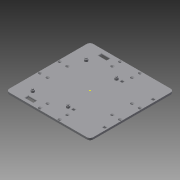
# Autodesk Inventor part: toppart
Saved by Autodesk Inventor 2015 (Build 190159000, 159)
## iProperties
Created: 2015-11-30
Part Number: toppart
Material: Generic
Document SubType Name: Modeling
Designer: Ross
Density: 1 g/cm^3
Appearance: Default
Author: Ross
Autodesk Inventor part; units mm, degrees
sketch "Sketch1" plane through (0, 0, 0) normal (0, 1, 0) x (-1, 0, 0)
  line L0 (0, 65) -> (65, 65)
  line L1 (65, 65) -> (65, -65)
  line L2 (65, -65) -> (0, -65)
  line L3 (0, -65) -> (-65, -65)
  line L4 (-65, -65) -> (-65, 65)
  line L5 (-65, 65) -> (0, 65)
  point P0 (0, 0)
  dimension "d0" = 65
  dimension "d1" = 65
  dimension "d2" = 130
  dimension "d3" = 65
  constraints: 12 end point, 4 perpendicular, 2 point on line
  measures "d0" distance of point (0, 0) L0.start
  measures "d1" distance of L0.start L0.end
  measures "d2" distance of L0.end L1.end
  measures "d3" distance of L2.end L3.end
extrude "Extrusion1" add sketch "Sketch1" along normal blind 3
fillet "Fillet1" radius 5 4 edges at (-65, 1.5, 65) (65, 1.5, 65) (-65, 1.5, -65) (65, 1.5, -65)
sketch "Sketch6" plane through (0, 3, 0) normal (0, 1, 0) x (1, 0, 0)
  line L0 (60, 65) -> (-60, 65) projected
  line L1 (0, 65) -> (-18.3, 65)
  line L2 (-18.3, 65) -> (-18.3, 47)
  line L3 (0, 65) -> (18.3, 65)
  line L4 (18.3, 65) -> (18.3, 47)
  line L5 (18.3, 47) -> (-18.3, 47)
  line L6 (-18.3, 47) -> (-15.3, 47)
  line L7 (-15.3, 47) -> (-15.3, 50)
  line L8 (-15.3, 65) -> (-15.3, 62)
  line L9 (0, 65) -> (0, 47)
  circle A0 centre (-15.3, 62) radius 2.4
  circle A1 centre (-15.3, 50) radius 2.4
  circle A2 centre (15.3, 62) radius 2.4
  circle A3 centre (15.3, 50) radius 2.4
  point P0 (0, 0)
  dimension "d20" = 18.3
  dimension "d21" = 18
  dimension "d22" = 18.3
  dimension "d23" = 3
  dimension "d24" = 3
  dimension "d25" = 3
  dimension "d40" = 4.8
  dimension "d41" = 4.8
  constraints: 18 end point, 4 centre point, 4 point on line, 2 coincident, 2 midpoint, 2 perpendicular, 2 symmetric about line, 1 vertical, 2 other
  measures "d20" distance of L1.start L1.end
  measures "d21" distance of L1.end L2.end
  measures "d22" distance of L1.start L3.end
  measures "d23" distance of L2.end L6.end
  measures "d24" distance of L6.end L7.end
  measures "d25" distance of L8.start L8.end
  measures "d40" diameter of A0
  measures "d41" diameter of A1
extrude "Extrusion6" cut sketch "Sketch6" against normal blind 1.5 contours A0
sketch "Sketch9" plane through (-15.3, 1.5, -62) normal (0, 1, 0) x (1, 0, 0)
  circle A0 centre (0, 0) radius 1.25
  point P0 (15.3, -62)
  dimension "d44" = 2.5
  constraints: 1 centre point
  measures "d44" diameter of A0
extrude "Extrusion7" cut sketch "Sketch9" against normal blind 1.5
ref_plane "Work Plane1" through (-15.25, 0, 0) normal (1, 0, 0) x (0, 1, 0)
sketch "Sketch11" plane through (-15.25, 0, 0) normal (1, 0, 0) x (0, 1, 0)
  line L0 (3, -59.6) -> (3, -64.4) projected
  line L1 (3, -59.6) -> (1.5, -59.6)
  line L2 (1.5, -59.6) -> (1.5, -64.4) projected
  line L3 (3, -59.6) -> (1.5, -59.6) projected
  line L4 (1.5, -59.6) -> (1.5, -60.7474)
  line L5 (1.5, -60.75) -> (1.5, -63.25) projected
  line L6 (1.5, -60.75) -> (3, -59.6)
  point P0 (0, 0)
  constraints: 8 end point, 1 collinear, 1 point on line
sketch3d "3D Sketch1"
  arc A0 (-12.9, 3, -62) -> (-15.3, 3, -59.6) centre (-15.3, 3, -62) ccw
  arc A1 (-15.3, 3, -59.6) -> (-17.7, 3, -62) centre (-15.3, 3, -62) ccw
  arc A2 (-17.7, 3, -62) -> (-15.3, 3, -64.4) centre (-15.3, 3, -62) ccw
  arc A3 (-15.3, 3, -64.4) -> (-12.9, 3, -62) centre (-15.3, 3, -62) ccw
sweep "Sweep1" add profiles "Sketch11" path "3D Sketch1"
ref_plane "Work Plane2" through (60, 0, -56) normal (0, 0, -1) x (-1, 0, 0)
ref_plane "Work Plane3" through (0, 0, -60) normal (-1, 0, 0) x (0, 0, 1)
mirror "Mirror5" about plane through (0, 0, -60) normal (-1, 0, 0) of "Extrusion7", "Sweep1"
mirror "Mirror6" about plane through (0, 0, -60) normal (-1, 0, 0) of "Extrusion6", "Extrusion7", "Sweep1"
mirror "Mirror7" about plane through (60, 0, -56) normal (0, 0, -1) of "Extrusion6", "Extrusion7", "Sweep1", "Mirror6"
pattern_circular "Circular Pattern3" count 4 over 360 about axis through (0, -10, 0) along (0, 1, 0) of "Extrusion6", "Extrusion7", "Sweep1", "Mirror6", "Mirror7"
sketch "Sketch14" plane through (0, 3, 0) normal (0, 1, 0) x (1, 0, 0)
  line L0 (65, -60) -> (10, -60)
  line L1 (10, -60) -> (10, 65)
  line L2 (-60, 65) -> (60, 65) projected
  line L3 (10, -60) -> (-44, -60)
  line L4 (-44, -60) -> (-44, 65)
  line L5 (37.5, -60) -> (37.5, 65)
  line L6 (37.5, -60) -> (14.5, -60)
  line L7 (14.5, -60) -> (14.5, 65)
  line L8 (60.5, -60) -> (60.5, 65)
  line L9 (65, -60) -> (65, 60) projected
  line L10 (59, -39.0209) -> (62, -39.0209)
  line L11 (62, -39.0209) -> (59, -39.0209)
  line L12 (59, -39.0209) -> (59, -36.0209)
  line L13 (59, -36.0209) -> (62, -36.0209)
  line L14 (62, -36.0209) -> (62, -39.0209)
  point P0 (0, 0)
  dimension "d56" = 55
  dimension "d57" = 54
  dimension "d58" = 23
  dimension "d63" = 3
  dimension "d64" = 3
  constraints: 26 end point, 5 point on line, 4 perpendicular, 3 horizontal, 2 parallel, 2 symmetric about line, 1 midpoint, 1 vertical
  measures "d56" distance of L0.start L0.end
  measures "d57" distance of L0.end L3.end
  measures "d58" distance of L5.start L6.end
  measures "d63" distance of L12.end L13.end
  measures "d64" distance of L11.end L12.end
extrude "Extrusion8" cut sketch "Sketch14" against normal blind 3 contours L10 L12 L13 L8 | L8 L13 L14 L10
fillet "Fillet2" radius 1 4 edges at (62, 3, 37.5209) (60.5, 3, 39.0209) (59, 3, 37.5209) (60.5, 3, 36.0209)
fillet "Fillet3" radius 2 1 edges at (59, 0, 37.5209)
ref_plane "Work Plane4" through (36.5, 0, -60) normal (-1, 0, 0) x (0, 0, 1)
mirror "Mirror8" about plane through (36.5, 0, -60) normal (-1, 0, 0) of "Extrusion8", "Fillet2", "Fillet3"
sketch "Sketch15" plane through (0, 3, 0) normal (0, 1, 0) x (1, 0, 0)
  point P0 (0, 0)
mirror "Mirror9" about plane through (0, 0, 0) normal (0, 0, 1) of "Fillet2", "Extrusion8", "Fillet3", "Mirror8"
sketch "Sketch16" plane through (0, 3, 0) normal (0, 1, 0) x (1, 0, 0)
  line L0 (63, -60) -> (11, -60)
  line L1 (11, -60) -> (11, 53.4976)
  line L2 (11, 53.4976) -> (63, 53.4976)
  line L3 (63, 53.4976) -> (63, -60)
  line L4 (9.645, 0) -> (9.645, -52)
  line L5 (9.645, -52) -> (-44.355, -52)
  line L6 (-44.355, -52) -> (-44.355, 50)
  line L7 (-44.355, 50) -> (9.645, 50)
  line L8 (9.645, 50) -> (9.645, -52)
  line L9 (-40.3154, -54.1219) -> (-28.3154, -54.1219)
  line L10 (-28.3154, -54.1219) -> (-28.3154, -59.1219)
  line L11 (-28.3154, -59.1219) -> (-40.3154, -59.1219)
  line L12 (-40.3154, -59.1219) -> (-40.3154, -54.1219)
  point P0 (0, 0)
  dimension "d70" = 52
  dimension "d71" = 52
  dimension "d72" = 54
  dimension "d73" = 102
  dimension "d74" = 12
  dimension "d75" = 5
  constraints: 26 end point, 6 parallel, 3 horizontal, 3 perpendicular, 1 vertical
  measures "d70" distance of L1.end L2.end
  measures "d71" distance of L4.start L4.end
  measures "d72" distance of L6.end L7.end
  measures "d73" distance of L5.end L6.end
  measures "d74" distance of L10.end L11.end
  measures "d75" distance of L9.end L10.end
extrude "Extrusion9" cut sketch "Sketch16" against normal blind 3 contours L9 L10 L11 L12
fillet "Fillet4" radius 1.5 4 edges at (-34.3154, 3, 59.1219) (-34.3154, 3, 54.1219) (-40.3154, 3, 56.6219) (-28.3154, 3, 56.6219)
fillet "Fillet5" radius 1.5 4 edges at (-34.3154, 0, 54.1219) (-28.3154, 0, 56.6219) (-34.3154, 0, 59.1219) (-40.3154, 0, 56.6219)
mirror "Mirror10" about plane through (0, 0, 0) normal (0, 0, 1) of "Extrusion9", "Fillet4", "Fillet5"
sketch "Sketch17" plane through (0, 3, 0) normal (0, 1, 0) x (1, 0, 0)
  line L0 (0, 0) -> (8, 0)
  line L1 (8, 0) -> (8, -50.76)
  line L2 (8, 0) -> (8, 50.76)
  line L3 (8, 50.76) -> (-45.3, 50.76)
  line L4 (-45.3, 50.76) -> (-45.3, -50.76)
  line L5 (-45.3, -50.76) -> (8, -50.76)
  line L6 (8, 50.76) -> (8, 35.52)
  line L7 (8, 35.52) -> (5.46, 35.52)
  circle A0 centre (5.46, 35.52) radius 2.5
  line L8 (-45.3, 50.76) -> (-45.3, 36.79)
  line L9 (-45.3, 36.79) -> (-42.76, 36.79)
  circle A1 centre (-42.76, 36.79) radius 2.5
  line L10 (8, 50.76) -> (8, -39.41)
  line L11 (8, -39.41) -> (5.46, -39.41)
  circle A2 centre (5.46, -39.41) radius 2.5
  line L12 (-45.3, 50.76) -> (-45.3, -45.76)
  line L13 (-45.3, -45.76) -> (-42.76, -45.76)
  circle A3 centre (-42.76, -45.76) radius 2.5
  dimension "d80" = 8
  dimension "d81" = 50.76
  dimension "d82" = 50.76
  dimension "d83" = 53.3
  dimension "d84" = 15.24
  dimension "d85" = 2.54
  dimension "d86" = 5
  dimension "d87" = 13.97
  dimension "d88" = 2.54
  dimension "d89" = 5
  dimension "d90" = 90.17
  dimension "d91" = 2.54
  dimension "d92" = 5
  dimension "d93" = 96.52
  dimension "d94" = 2.54
  dimension "d95" = 5
  constraints: 28 end point, 6 perpendicular, 4 centre point, 4 coincident, 4 point on line, 2 vertical, 1 horizontal, 1 parallel
  measures "d80" distance of L0.start L0.end
  measures "d81" distance of L0.end L1.end
  measures "d82" distance of L0.end L2.end
  measures "d83" distance of L2.end L3.end
  measures "d84" distance of L2.end L6.end
  measures "d85" distance of L6.end L7.end
  measures "d86" diameter of A0
  measures "d87" distance of L3.end L8.end
  measures "d88" distance of L8.end L9.end
  measures "d89" diameter of A1
  measures "d90" distance of L2.end L10.end
  measures "d91" distance of L10.end L11.end
  measures "d92" diameter of A2
  measures "d93" distance of L3.end L12.end
  measures "d94" distance of L12.end L13.end
  measures "d95" diameter of A3
extrude "Extrusion10" add sketch "Sketch17" along normal blind 3 contours A0 | A1 | A2 | A3
sketch "Sketch18" plane through (-42.76, 6, -36.79) normal (0, 1, 0) x (1, 0, 0)
  circle A0 centre (0, 0) radius 2.5 projected
  circle A1 centre (0, 0) radius 1.5
  point P0 (42.76, -36.79)
  dimension "d98" = 3
  constraints: 1 centre point, 1 coincident
  measures "d98" diameter of A1
extrude "Extrusion11" add sketch "Sketch18" along normal blind 1.5 contours A1
sketch "Sketch19" plane through (5.46, 6, -35.52) normal (0, 1, 0) x (1, 0, 0)
  circle A0 centre (0, 0) radius 2.5 projected
  circle A1 centre (0, 0) radius 1.5
  point P0 (-5.46, -35.52)
  dimension "d101" = 3
  constraints: 1 centre point, 1 coincident
  measures "d101" diameter of A1
extrude "Extrusion12" add sketch "Sketch19" along normal blind 1.5 contours A1
sketch "Sketch20" plane through (5.46, 6, 39.41) normal (0, 1, 0) x (1, 0, 0)
  circle A0 centre (0, 0) radius 1.5
  point P0 (-5.46, 39.41)
  dimension "d104" = 3
  constraints: 1 centre point
  measures "d104" diameter of A0
extrude "Extrusion13" add sketch "Sketch20" along normal blind 1.5
sketch "Sketch21" plane through (-42.76, 6, 45.76) normal (0, 1, 0) x (1, 0, 0)
  circle A0 centre (0, 0) radius 1.5
  point P0 (42.76, 45.76)
  dimension "d107" = 3
  constraints: 1 centre point
  measures "d107" diameter of A0
extrude "Extrusion14" add sketch "Sketch21" along normal blind 1.5
fillet "Fillet6" radius 0.5 1 edges at (-44.26, 7.5, 45.76)
fillet "Fillet7" radius 0.5 3 edges at (3.96, 7.5, 39.41) (3.96, 7.5, -35.52) (-44.26, 7.5, -36.79)
body "Solid1"
